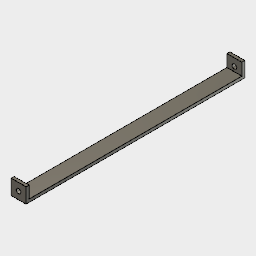
Untitled v1 (Autodesk Fusion 360 design; units mm, degrees)
Autodesk Fusion 360 part; units mm, degrees
note: some values were not read from the file. Set by a fixed rule: which sketch regions a step uses.
sketch "Sketch1" plane through (0, 0, 0) normal (0, 0, 1) x (1, 0, 0)
  line L0 (-14.9621, 7.481) -> (-4.9621, 7.481)
  line L1 (-4.9621, 7.481) -> (-4.9621, -2.519)
  line L2 (-4.9621, -2.519) -> (-14.9621, -2.519)
  line L3 (-14.9621, -2.519) -> (-14.9621, 7.481)
  line L4 (-14.9621, 7.481) -> (-9.9621, 7.481)
  line L5 (-14.9621, 7.481) -> (-9.9621, 7.481)
  line L6 (-9.9621, 7.481) -> (-9.9621, 2.481)
  line L7 (-4.9621, 7.481) -> (-9.9621, 7.481)
  circle A0 centre (-9.9621, 2.481) radius 1.5
  dimension "d1" = 10
  dimension "d2" = 10
  dimension "d3" = 5
  dimension "d4" = 3
  measures "d1" distance of L0.start L0.end
  measures "d2" distance of L0.start L2.end
  measures "d3" distance of L4.end L6.end
  measures "d4" diameter of A0
extrude "Extrude1" add sketch "Sketch1" along normal blind 2
sketch "Sketch2" plane through (0, 0, 2) normal (0, 0, 1) x (1, 0, 0)
  circle A0 centre (-9.9621, 2.481) radius 1.5
  line L0 (-4.9621, -2.519) -> (-4.9621, 7.481)
  line L1 (-4.9621, 7.481) -> (-14.9621, 7.481)
  line L2 (-14.9621, 7.481) -> (-14.9621, -2.519)
  line L3 (-14.9621, -2.519) -> (-4.9621, -2.519)
  line L4 (-14.9621, -2.519) -> (-4.9621, -2.519)
  line L5 (-4.9621, -2.519) -> (-4.9621, -0.519)
  line L6 (-4.9621, -0.519) -> (-14.9621, -0.519)
  line L7 (-14.9621, -0.519) -> (-14.9621, -2.519)
  dimension "d7" = 10
  dimension "d8" = 2
  measures "d7" distance of L2.end L0.start
  measures "d8" distance of L2.end L6.end
extrude "Extrude2" add sketch "Sketch2" along normal blind 5 contours L0 L2 L3 L4 L5 L6 L7
extrude "Extrude3" add 1 faces at (-11.6287, -1.8523, 7) along direction (0, 0, 1) blind 136
sketch "Sketch3" plane through (0, 0, 143) normal (0, 0, 1) x (1, 0, 0)
  line L0 (-14.9621, -0.519) -> (-14.9621, -2.519)
  line L1 (-14.9621, -2.519) -> (-4.9621, -2.519)
  line L2 (-4.9621, -2.519) -> (-4.9621, -0.519)
  line L3 (-4.9621, -0.519) -> (-14.9621, -0.519)
  line L4 (-14.9621, -2.519) -> (-4.9621, -2.519)
  line L5 (-4.9621, -2.519) -> (-4.9621, 7.481)
  line L6 (-4.9621, 7.481) -> (-14.9621, 7.481)
  line L7 (-14.9621, 7.481) -> (-14.9621, -2.519)
  line L8 (-14.9621, -2.519) -> (-9.9621, -2.519)
  line L9 (-9.9621, -2.519) -> (-9.9621, 2.481)
  circle A0 centre (-9.9621, 2.481) radius 1.5
  dimension "d13" = 10
  dimension "d14" = 10
  dimension "d15" = 5
  dimension "d16" = 3
  measures "d13" distance of L0.end L1.end
  measures "d14" distance of L0.end L6.end
  measures "d15" distance of L8.end L9.end
  measures "d16" diameter of A0
extrude "Extrude4" add sketch "Sketch3" along normal blind 2
